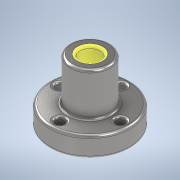
# Autodesk Inventor part: Gehaeuselager_8mm
Saved by Autodesk Inventor 2021 (Build 250183000, 183)
## iProperties
Created: 2021-04-16
Part Number: Gehaeuselager_8mm
Material: Generic
Document SubType Name: Modeling
Designer: Fabijan_Sven
Density: 1 g/cm^3
Appearance: Galvanized
Author: Fabijan_Sven
Autodesk Inventor part; units mm, degrees
ref_plane "YZ Plane" through (0, 0, 0) normal (1, 0, 0) x (0, 1, 0)
ref_plane "XZ Plane" through (0, 0, 0) normal (0, 1, 0) x (-1, 0, 0)
ref_plane "XY Plane" through (0, 0, 0) normal (0, 0, 1) x (1, 0, 0)
sketch "Sketch1" plane through (0, 0, 0) normal (0, 1, 0) x (-1, 0, 0)
  circle A0 centre (0, 0) radius 16
  circle A1 centre (0, 0) radius 4
  dimension "d0" = 32
  dimension "d1" = 8
  constraints: 2 centre point, 2 coincident
  measures "d0" diameter of A0
  measures "d1" diameter of A1
extrude "Extrusion1" add sketch "Sketch1" along normal blind 8
sketch "Sketch2" plane through (0, 8, 0) normal (0, 1, 0) x (1, 0, 0)
  circle A0 centre (0, 0) radius 4
  circle A1 centre (0, 0) radius 8
  dimension "d4" = 16
  dimension "d5" = 8
  constraints: 2 centre point, 2 coincident
  measures "d4" diameter of A1
  measures "d5" diameter of A0
extrude "Extrusion2" add sketch "Sketch2" along normal blind 17
sketch "Sketch3" plane through (0, 8, 0) normal (0, 1, 0) x (1, 0, 0)
  circle A0 centre (12, 0) radius 1.75
  circle A1 centre (0, 12) radius 1.75
  circle A2 centre (-12, 0) radius 1.75
  circle A3 centre (0, -12) radius 1.75
  line L0 (0, -17.2279) -> (0, 18.5252) construction
  line L1 (18.42, 0) -> (-19.0524, 0) construction
  point P0 (0, 0)
  dimension "d8" = 12
  dimension "d9" = 12
  dimension "d10" = 12
  dimension "d11" = 12
  dimension "d12" = 3.5
  dimension "d13" = 3.5
  dimension "d14" = 3.5
  dimension "d15" = 3.5
  constraints: 4 centre point, 4 end point, 4 point on line, 1 horizontal, 1 vertical
  measures "d8" distance of A1.centre point (0, 0)
  measures "d9" distance of point (0, 0) A2.centre
  measures "d10" distance of A3.centre point (0, 0)
  measures "d11" distance of A0.centre point (0, 0)
  measures "d12" diameter of A2
  measures "d13" diameter of A1
  measures "d14" diameter of A0
  measures "d15" diameter of A3
extrude "Extrusion3" cut sketch "Sketch3" against normal blind 20
fillet "Fillet1" radius 1 6 edges at (16, 8, 0) (16, 0, 0) (-4, 25, 0) (-8, 25, 0) (-8, 8, 0) (4, 0, 0)
fillet "Fillet2" radius 1 8 edges at (-13.75, 8, 0) (-1.75, 8, 12) (10.25, 8, 0) (-1.75, 8, -12) (-1.75, 0, 12) (10.25, 0, 0) (-1.75, 0, -12) (-13.75, 0, 0)
body "Solid1"
